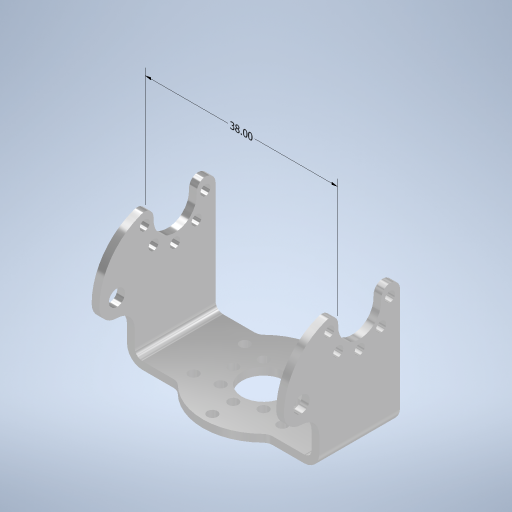
# Autodesk Inventor part: sholder
Saved by Autodesk Inventor 2024.1 (Build 281209000, 209)
## iProperties
Created: 2024-02-14
Part Number: sholder
Material: アルミニウム 6061
Document SubType Name: Sheet Metal
Designer: hibik
Density: 2.7 g/cm^3
Sheet Metal Rule: Default_mm
Appearance: アルミニウム - フラット
Flat Pattern Width: 2.7 cm
Flat Pattern Length: 8.34605 cm
Flat Pattern Area: 22.5343 cm^2
Sheet Metal Width: 27.000 mm
Sheet Metal Length: 83.461 mm
Sheet Metal Area: 2253.434 mm^2
Author: hibik
Autodesk Inventor part; units mm, degrees
ref_plane "YZ Plane" through (0, 0, 0) normal (1, 0, 0) x (0, 1, 0)
ref_plane "XZ Plane" through (0, 0, 0) normal (0, 1, 0) x (-1, 0, 0)
ref_plane "XY Plane" through (0, 0, 0) normal (0, 0, 1) x (1, 0, 0)
sketch "スケッチ1" plane through (0, 0, 0) normal (0, 1, 0) x (-1, 0, 0)
  line L0 (19, 8) -> (-19, 8)
  line L1 (-19, 8) -> (-19, -8)
  line L2 (-19, -8) -> (19, -8)
  line L3 (19, -8) -> (19, 8)
  line L4 (19, 8) -> (-19, -8) construction
  line L5 (-19, 8) -> (19, -8) construction
  circle A0 centre (0, 0) radius 4.25
  circle A1 centre (0, 0) radius 6
  circle A2 centre (0, 6) radius 1
  line L6 (0, -16.8) -> (0, 16.8)
  circle A3 centre (-4.2426, 4.2426) radius 1
  circle A4 centre (-6, 0) radius 1
  circle A5 centre (-4.2426, -4.2426) radius 1
  circle A6 centre (0, -6) radius 1
  circle A7 centre (4.2426, -4.2426) radius 1
  circle A8 centre (0, 0) radius 12
  circle A9 centre (6, 0) radius 1
  circle A10 centre (4.2426, 4.2426) radius 1
  point P0 (-8.9443, -8)
  point P1 (8.9443, -8)
  point P2 (-8.9443, 8)
  point P3 (8.9443, 8)
  dimension "d1" = 12
  dimension "d0" = 8.5
  dimension "d2" = 2
  dimension "d5" = 360
  dimension "d8" = 16
  dimension "d9" = 38
  dimension "d21" = 24
  measures "d0" diameter of A0
  measures "d2" diameter of A2
  measures "d8" distance of L2.end L0.start
  measures "d9" distance of L0.start L0.end
  measures "d21" diameter of A8
extrude "プレート1" add sketch "スケッチ1" along normal blind 1.5 contours L3 L2 A8 L0 | A8 L2 L6 A6 A1 A7 A9 A10 A2 L0 | L0 L6 A8 | L6 A2 A1 A3 A4 A5 A6 L2 A8 L0 | L0 A8 L6 | A8 L6 L2 | A8 L2 L1 L0 | L6 A8 L2 | A2 L6 A0 A6 A1 A5 A4 A3 | A1 A10 A9 A7 A6 L6 A0 A2
sketch "スケッチ2" plane through (-17.5, 0, 8) normal (-1, 0, 0) x (0, -1, 0)
  line L0 (0, -16) -> (0, 0)
  line L1 (0, 0) -> (-30, 0)
  line L2 (-30, 0) -> (-30, -16)
  line L3 (-30, -16) -> (0, -16)
  constraints: 6 end point, 1 horizontal, 1 perpendicular, 1 vertical
edge flange "フランジ1" height 30 angle 90 thickness 1.5 bend radius 1.5 thickness toward (-1, 0, 0) relief straight relief width 1.5 relief depth 0.75 corner gap 1.5 corner form 0 edges at (-19, 1.5, 0) (19, 1.5, 0) wall of the first edge with corners at (-17.5, 0, -8) (-17.5, 0, 8) (-17.5, 30, 8) (-17.5, 30, -8)
bend "曲げ1"
corner "コーナー1"
sketch "スケッチ3" plane through (0, 1.5, 0) normal (0, 1, 0) x (1, 0, 0)
  circle A0 centre (8.7685, -5.0625) radius 1 projected
  circle A1 centre (8.7685, 5.0625) radius 1 projected
  circle A2 centre (0, 10.125) radius 1 projected
  circle A3 centre (-8.7685, 5.0625) radius 1 projected
  circle A4 centre (-8.7685, -5.0625) radius 1 projected
  circle A5 centre (0, -10.125) radius 1 projected
  point P0 (0, 0)
extrude "切り取り1" cut sketch "スケッチ3" against normal blind 1.5
sketch "スケッチ4" plane through (19, 30, 8) normal (1, 0, 0) x (0, 0, -1)
  circle A0 centre (8, -7) radius 4.25
  line L0 (0, -27) -> (16, -27) projected
  circle A1 centre (8, -7) radius 6 construction
  circle A2 centre (8, -13) radius 1
  circle A3 centre (12.2426, -11.2426) radius 1
  circle A4 centre (14, -7) radius 1
  circle A5 centre (12.2426, -2.7574) radius 1
  circle A6 centre (8, -1) radius 1
  circle A7 centre (3.7574, -2.7574) radius 1
  line L1 (16, -27) -> (16, 0) projected
  line L2 (0, 0) -> (16, 0)
  line L3 (16, 0) -> (16, -7)
  line L4 (16, -7) -> (0, -7)
  line L5 (0, -7) -> (0, 0)
  line L6 (0, 0) -> (16, 0) projected
  circle A8 centre (2, -7) radius 1
  circle A9 centre (3.7574, -11.2426) radius 1
  line L7 (8, -7) -> (16, -3.6863)
  line L8 (8, -7) -> (0, -3.6863)
  line L9 (2, -7) -> (3.7574, -2.7574)
  line L10 (12.2426, -2.7574) -> (14, -7)
  point P0 (8, -30)
  point P1 (8, -27)
  point P2 (8, -27)
  point P3 (13.1213, -4.8787)
  point P4 (2.8787, -4.8787)
  dimension "d24" = 20
  dimension "d25" = 8.5
  dimension "d26" = 12
  dimension "d27" = 2
  dimension "d30" = 360
  constraints: 16 end point, 10 centre point, 5 midpoint, 5 point on line, 4 coincident, 2 parallel, 2 point on circle, 2 vertical alignment, 1 collinear, 1 horizontal, 1 perpendicular, 23 other
  measures "d24" distance from line of L0 A0.centre
  measures "d25" diameter of A0
  measures "d26" diameter of A1
  measures "d27" diameter of A2
extrude "切り取り2" cut sketch "スケッチ4" against normal blind 38 contours L4 L7 A0 | A0 L4 | L7 L8 A0 | A6 | A0 L8 L5 L2 L1 L7 | A0 L8 L4 | L4 A4 | A4 L10 L4 | A8 L4 | L4 L9 A8 | A4 L4 L10 | L4 A8 L9 | A2 | A3 | A5 | A7 | A9
fillet "フィレット1" radius 2 12 edges at (-8.9443, 0.75, 8) (8.9443, 0.75, 8) (8.9443, 0.75, -8) (-8.9443, 0.75, -8) (18.25, 24.6264, 3.9265) (18.25, 24.6264, -3.9265) (-18.25, 24.6264, 3.9265) (-18.25, 24.6264, -3.9265) (18.25, 26.3137, 8) (18.25, 26.3137, -8) (-18.25, 26.3137, -8) (-18.25, 26.3137, 8)
sketch "スケッチ6" plane through (19, 3, 8) normal (1, 0, 0) x (0, 0, -1)
  circle A0 centre (-3.5, 10.3373) radius 1.6
  circle A1 centre (-3.5, 10.3373) radius 3.5
  line L0 (0, 0) -> (0, 20.3373)
  arc A2 (2.5294, 22.266) -> (0, 20.3373) centre (2, 20.3373) ccw
  arc A3 (1.3154, 22.2165) -> (-7, 10.3373) centre (5.6429, 10.3373) ccw
  line L1 (0, -1.5) -> (0, 0)
  arc A4 (0, 3.3373) -> (-3.5, 6.8373) centre (-3.5, 3.3373) ccw
  point P0 (8, -3)
  point P1 (0, -0.75)
  dimension "d35" = 3.2
  dimension "d36" = 7
  dimension "d38" = 10
  measures "d35" diameter of A0
  measures "d36" diameter of A1
  measures "d38" vertical distance of A2.centre A0.centre
sheet face with bend "面2" sketch "スケッチ6" thickness 1.5 toward (-1, 0, 0) bend radius 1.5 relief straight relief width 1.5 relief depth 0.75
bend "曲げ2"
mirror "ミラー1" about plane through (0, 0, 0) normal (1, 0, 0) of "面2"
equation "\"d22\" = Thickness"
equation "\"d10\" = Thickness"
equation "\"d11\" = BendReliefWidth"
equation "\"d12\" = BendReliefDepth"
equation "\"d13\" = MinimumRemnant"
equation "\"d14\" = TransitionRadius"
equation "\"d17\" = BendRadius"
equation "\"d18\" = CornerReliefSize"
equation "\"d19\" = GapSize"
equation "\"d20\" = JacobiRadiusSize"
equation "\"d39\" = BendRadius"
equation "\"d40\" = BendReliefWidth"
equation "\"d42\" = MinimumRemnant"
equation "\"d41\" = BendReliefDepth"
equation "\"d43\" = TransitionRadius"
equation "\"BendRadius\" = Thickness"
equation "\"BendReliefWidth\" = Thickness"
equation "\"BendReliefDepth\" = 0.5 * Thickness"
equation "\"CornerReliefSize\" = 4 * Thickness"
equation "\"MinimumRemnant\" = 2 * Thickness"
equation "\"TransitionRadius\" = BendRadius"
equation "\"GapSize\" = Thickness"
equation "\"Thickness\" = 1.5"
equation "\"JacobiRadiusSize\" = 1.5"
